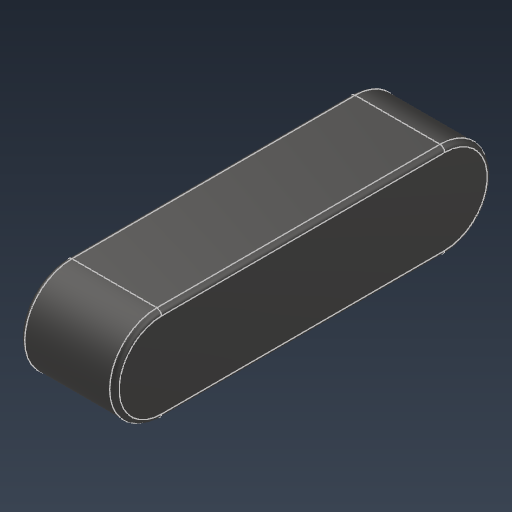
# Autodesk Inventor part: MCEN4000:G3K
Saved by Autodesk Inventor 2021 (Build 250183000, 183)
## iProperties
Created: 2020-10-20
Part Number: MCEN4000:G3K
Material: STEEL, AISI 1015
Document SubType Name: Modeling
Designer: Eugene Tang
Density: 7.85 g/cm^3
Appearance: AISI 1015
Mass: 3.70487 g
Surface Area: 4.07945 cm^2
Volume: 0.471958 cm^3
Description: PINION KEY (DIN 6885)
PKey_W: 5.000 mm
Author: Eugene Tang
Autodesk Inventor part; units mm, degrees
ref_plane "YZ Plane" through (0, 0, 0) normal (1, 0, 0) x (0, 1, 0)
ref_plane "XZ Plane" through (0, 0, 0) normal (0, 1, 0) x (-1, 0, 0)
ref_plane "XY Plane" through (0, 0, 0) normal (0, 0, 1) x (1, 0, 0)
sketch "Sketch1" plane through (0, 0, 0) normal (0, 0, 1) x (1, 0, 0)
  line L0 (-2.5, 2.5) -> (2.5, 2.5)
  line L1 (2.5, 2.5) -> (2.5, -2.5)
  line L2 (2.5, -2.5) -> (-2.5, -2.5)
  line L3 (-2.5, -2.5) -> (-2.5, 2.5)
  line L4 (-3.5, 0) -> (3.5, 0) construction
  line L5 (0, -3.5) -> (0, 3.5) construction
  point P0 (0, 0)
  point P1 (-2.5, 0)
  point P2 (0, -2.5)
  dimension "PKey_W" = 5
  constraints: 8 end point, 2 midpoint, 2 parallel, 2 perpendicular, 2 point on line, 1 horizontal
  measures "PKey_W" distance between parallel lines of L3 L1
extrude "Extrusion1" add sketch "Sketch1" against normal blind 20
full round fillet "Fillet2" first side at (-0.8333, -2.5, -6.6667) centre faces at (-0.8333, -0.8333, 0) second side at (0.8333, 2.5, -6.6667)
full round fillet "Fillet3" first side at (0.8333, -2.5, -14.1666) centre faces at (-0.8333, -0.8333, -20) second side at (-0.8333, 2.5, -14.1666)
fillet "Fillet1" radius 0.25 4 edges at (-2.5, 2.5, -10) (-2.5, -2.5, -10) (2.5, 2.5, -10) (2.5, -2.5, -10)
equation "\"d1\" = PinionKey_L"
equation "\"TD\" = 0.3"
equation "\"Ball_DIA\" = 6"
equation "\"Screw_L\" = 292"
equation "\"Screw_DIA\" = 36"
equation "\"Nut_OD\" = 66"
equation "\"BPath_REVQ\" = 5.75"
equation "\"Tread_OFFSET\" = 8.075"
equation "\"SteeringColumn_DIA\" = 26"
equation "\"SteeringColumnChamfer_DEG\" = 20deg"
equation "\"Rack_L\" = 307.252"
equation "\"NutCapTread_L\" = 25"
equation "\"NutCapTread_THICKNESS\" = 5.365"
equation "\"SupportFlange_THICKNESS\" = 5"
equation "\"GearKey_L\" = 32"
equation "\"PinionKey_L\" = 20"
body "Solid1"
